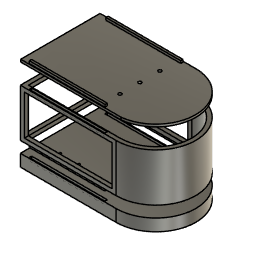
Modele3D_FusionAutodesk (Autodesk Fusion 360 design; units mm, degrees)
Autodesk Fusion 360 part; units mm, degrees
note: some values were not read from the file. Chosen so that the rebuilt part matches the saved one: which bodies a step acts on.
sketch "Esquisse1" plane through (0, 0, 0) normal (0, 0, 1) x (1, 0, 0)
  line L0 (0, 0) -> (120, 0)
  line L1 (120, 100) -> (0, 100)
  line L2 (0, 100) -> (0, 0)
  arc A0 (120, 0) -> (120, 100) centre (120, 50) ccw
  dimension "d1" = 120
  dimension "d2" = 100
  constraint horizontal L0
  constraint horizontal L1
  constraint vertical L2
  constraint coincident L0.start L2.end
  measures "d1" distance of L0.start L0.end
  measures "d2" distance of L0.start L1.end
extrude "Extrusion1" add sketch "Esquisse1" along normal blind 5 makes body 1
sketch "Esquisse2" plane through (0, 0, 5) normal (0, 0, 1) x (-1, 0, 0)
  arc A0 (-120, 0) -> (-120, -100) centre (-120, -50) ccw
  line L0 (-120, -100) -> (0, -100)
  line L1 (0, -100) -> (0, 0)
  line L2 (0, 0) -> (-120, 0)
  line L3 (-5, -95) -> (-120, -95)
  line L4 (-120, -5) -> (-5, -5)
  line L5 (-5, -5) -> (-5, -95)
  arc A1 (-120, -5) -> (-120, -95) centre (-120, -50) ccw
  dimension "d7" = 90
  constraint horizontal L3
  constraint horizontal L4
  constraint vertical L5
  constraint concentric A0 A1
  measures "d7" diameter of A1
extrude "Extrusion2" add sketch "Esquisse2" along normal blind 60 separate body makes body 2
sketch "Esquisse3" plane through (0, 0, 0) normal (0, -1, 0) x (1, 0, 0)
  line L0 (0, 5) -> (120, 5)
  line L1 (120, 5) -> (120, 65)
  line L2 (120, 65) -> (0, 65)
  line L3 (0, 65) -> (0, 5)
  line L4 (5, 60) -> (115, 60)
  line L5 (115, 60) -> (115, 10)
  line L6 (115, 10) -> (5, 10)
  line L7 (5, 10) -> (5, 60)
  constraint horizontal L4
  constraint vertical L5
  constraint horizontal L6
  constraint vertical L7
extrude "Extrusion3" cut sketch "Esquisse3" against normal blind 30 contours L4 L5 L6 L7 picked at (41.666667, 43.333333) bodies 2
sketch "Esquisse4" plane through (0, 0, 0) normal (-1, 0, 0) x (0, -1, 0)
  line L0 (-100, 5) -> (0, 5)
  line L1 (0, 5) -> (0, 65)
  line L2 (0, 65) -> (-100, 65)
  line L3 (-100, 65) -> (-100, 5)
  line L4 (-95, 60) -> (-5, 60)
  line L5 (-5, 60) -> (-5, 10)
  line L6 (-5, 10) -> (-95, 10)
  line L7 (-95, 10) -> (-95, 60)
  line L8 (-95, 60) -> (-5, 60)
  line L9 (-5, 60) -> (-5, 10)
  line L10 (-5, 10) -> (-95, 10)
  line L11 (-95, 10) -> (-95, 60)
  constraint horizontal L4
  constraint vertical L5
  constraint horizontal L6
  constraint vertical L7
  constraint horizontal L8
  constraint vertical L9
  constraint horizontal L10
  constraint vertical L11
extrude "Extrusion4" cut sketch "Esquisse4" against normal blind 30 contours L4 L5 L6 L7 L8 L9 L10 L11 picked at (-65, 43.333333) bodies 2
sketch "Esquisse5" plane through (0, 100, 0) normal (0, 1, 0) x (-1, 0, 0)
  line L0 (-120, 5) -> (0, 5)
  line L1 (0, 5) -> (0, 65)
  line L2 (0, 65) -> (-120, 65)
  line L3 (-120, 65) -> (-120, 5)
  line L4 (-115, 60) -> (-5, 60)
  line L5 (-5, 60) -> (-5, 10)
  line L6 (-5, 10) -> (-115, 10)
  line L7 (-115, 10) -> (-115, 60)
  constraint horizontal L4
  constraint vertical L5
  constraint horizontal L6
  constraint vertical L7
extrude "Extrusion5" cut sketch "Esquisse5" against normal blind 30 contours L4 L5 L6 L7 picked at (-78.333333, 43.333333) bodies 2
sketch "Esquisse6" plane through (0, 0, 65) normal (0, 0, 1) x (-1, 0, 0)
  line L0 (-120, -5) -> (-5, -5)
  line L1 (-5, -5) -> (-5, -95)
  line L2 (-5, -95) -> (-120, -95)
  arc A0 (-120, -5) -> (-120, -95) centre (-120, -50) ccw
  line L3 (0, 0) -> (-120, 0)
  arc A1 (-120, 0) -> (-120, -100) centre (-120, -50) ccw
  line L4 (-120, -100) -> (0, -100)
  line L5 (0, -100) -> (0, 0)
  line L6 (-126.00428, -0.361823) -> (0, -0.361823)
  line L7 (0, -0.361823) -> (0, -100)
  line L8 (0, -100) -> (-126.00428, -100)
  arc A2 (-125.853995, -0.361823) -> (-126.00428, -99.620223) centre (-120, -50) ccw
  line L9 (-126.00428, -100) -> (-126.00428, -99.620223)
  line L10 (-126.00428, -0.379777) -> (-126.00428, -0.361823)
  constraint concentric A0 A2
  constraint horizontal L6
  constraint vertical L7
  constraint horizontal L8
  constraint vertical L9
  constraint collinear L9 L10
extrude "Extrusion6" add sketch "Esquisse6" along normal blind 3 separate body contours L0 L1 L2 A0 picked at (-43.333333, -65) makes body 3
extrude "Extrusion7" add sketch "Esquisse6" along normal blind 3 contours A1 L4 L5 L6 L7 L8 A2 picked at (-41.666667, -98.333333) bodies 2 3
extrude "Extrusion13" add sketch "Esquisse6" along normal blind 3 separate body contours L0 L1 L2 A0 picked at (-43.333333, -65) makes body 4
extrude "Extrusion14" add sketch "Esquisse6" along normal blind 3 separate body contours A1 L4 L5 L6 L7 L8 A2 picked at (-41.666667, -98.333333) makes body 5
sketch "Esquisse7" plane through (0, 0, 68) normal (0, 0, 1) x (-1, 0, 0)
  arc A0 (-125.853995, -0.361823) -> (-126.00428, -99.620223) centre (-120, -50) ccw
  line L0 (-126.00428, -99.620223) -> (-126.00428, -99.638177)
  arc A1 (-126.00428, -99.638177) -> (-120, -100) centre (-120, -50) ccw
  line L1 (-120, -100) -> (0, -100)
  line L2 (0, -100) -> (0, -0.361823)
  line L3 (0, -0.361823) -> (-125.853995, -0.361823)
  circle A2 centre (-100, -50) radius 2
  circle A3 centre (-100, -75) radius 2
  circle A4 centre (-100, -25) radius 2
  dimension "d37" = 4
  dimension "d38" = 4
  dimension "d39" = 4
  measures "d37" diameter of A2
  measures "d38" diameter of A3
  measures "d39" diameter of A4
extrude "Extrusion15" cut sketch "Esquisse7" against normal blind 3 contours A3 picked at (-99.58434, -74.280056) bodies 2 4
extrude "Extrusion16" cut sketch "Esquisse7" against normal blind 3 contours A2 picked at (-100.880609, -50.482818) bodies 2 4
extrude "Extrusion17" cut sketch "Esquisse7" against normal blind 3 contours A4 picked at (-100.975823, -25.453448) bodies 2 4
extrude "Extrusion18" cut sketch "Esquisse7" against normal blind 3 contours A4 picked at (-100.975823, -25.453448) bodies 2 4
sketch "Esquisse9" plane through (0, 0, 0) normal (0, 0, -1) x (1, 0, 0)
  arc A0 (120, -100) -> (120, 0) centre (120, -50) ccw
  line L0 (120, 0) -> (0, 0)
  line L1 (0, 0) -> (0, -100)
  line L2 (0, -100) -> (120, -100)
  circle A1 centre (25, -25) radius 1.15
  circle A2 centre (25, -75) radius 1.15
  circle A3 centre (48.65, -25) radius 1.15
  circle A4 centre (48.65, -75) radius 1.15
  point P0 (48.65, -25)
  point P1 (48.65, -75)
  dimension "d48" = 2.3
  dimension "d51" = 23.65
  dimension "d52" = 0
  dimension "d53" = 2.3
  dimension "d56" = 23.65
  dimension "d57" = 0
  dimension "d58" = 2.3
  dimension "d59" = 2.3
  constraint coincident P0 A3.centre
  constraint coincident P1 A4.centre
  measures "d48" diameter of A1
  measures "d53" diameter of A2
  measures "d58" diameter of A3
  measures "d59" diameter of A4
move_body "Déplacer1" bodies 1 to x (1, 0, 0) y (0, 1, 0) z (0, 0, 1) at (0, 0, -25)
sketch "Esquisse10" plane through (0, 0, 5) normal (0, 0, -1) x (1, 0, 0)
  line L0 (5, -5) -> (120, -5)
  arc A0 (120, -95) -> (120, -5) centre (120, -50) ccw
  line L1 (120, -95) -> (5, -95)
  line L2 (5, -95) -> (5, -5)
  line L3 (120, 0) -> (0, 0)
  line L4 (0, 0) -> (0, -100)
  line L5 (0, -100) -> (120, -100)
  arc A1 (120, -100) -> (120, 0) centre (120, -50) ccw
  line L6 (95.000001, -98.000001) -> (20, -98.000001)
  line L7 (20, -98.000001) -> (20, -97.000001)
  line L8 (20, -97.000001) -> (95.000001, -97.000001)
  line L9 (95.000001, -97.000001) -> (95.000001, -98.000001)
  constraint horizontal L6
  constraint vertical L7
  constraint horizontal L8
  constraint vertical L9
sketch "Esquisse11" plane through (0, 0, -20) normal (0, 0, 1) x (-1, 0, 0)
  arc A0 (-120, 0) -> (-120, -100) centre (-120, -50) ccw
  line L0 (-120, -100) -> (0, -100)
  line L1 (0, -100) -> (0, 0)
  line L2 (0, 0) -> (-120, 0)
move_body "Déplacer2" bodies 1 to x (1, 0, 0) y (0, 1, 0) z (0, 0, 1) at (0, 0, 25)
hole "Perçage1" at (48.634956, 74.989415, 0) direction (0, 0, 1) diameter 2.529 depth 8 tip angle 180 bodies 1
thread "Filetage1" "ISO Metric profile 3.0 M3x0.5 6H" thread offset 0 thread depth 7.4
hole "Perçage2" at (25, 75, 0) direction (0, 0, 1) diameter 2.529 depth 8 tip angle 180 bodies 1
thread "Filetage2" "ISO Metric profile 3.0 M3x0.5 6H" thread offset 0 thread depth 7.4
hole "Perçage3" at (25.005704, 24.988017, 0) direction (0, 0, 1) diameter 2.529 depth 8 tip angle 180 bodies 1
thread "Filetage3" "ISO Metric profile 3.0 M3x0.5 6H" thread offset 0 thread depth 7.4
hole "Perçage4" at (48.67047, 24.997067, 0) direction (0, 0, 1) diameter 2.529 depth 8 tip angle 180 bodies 1
thread "Filetage4" "ISO Metric profile 3.0 M3x0.5 6H" thread offset 0 thread depth 7.4
move_body "Déplacer3" bodies 1 to x (1, 0, 0) y (0, 1, 0) z (0, 0, 1) at (0, 0, -20)
extrude "Extrusion19" add 1 faces at (96.615853, 41.81968, -15) along direction (0, 0, 1) blind 10 on bodies 1 bodies 1
sketch "Esquisse12" plane through (0, 0, -20) normal (0, 0, -1) x (1, 0, 0)
  circle A0 centre (48.67047, -24.997067) radius 1.2645
  circle A1 centre (25.005704, -24.988017) radius 1.2645
  circle A2 centre (25, -75) radius 1.2645
  circle A3 centre (48.634956, -74.989415) radius 1.2645
  arc A4 (120, -100) -> (120, 0) centre (120, -50) ccw
  line L0 (120, 0) -> (0, 0)
  line L1 (0, 0) -> (0, -100)
  line L2 (0, -100) -> (120, -100)
  circle A5 centre (145.000002, -31) radius 1.25
  circle A6 centre (145.000002, -69.000001) radius 1.25
  line L3 (114.96183, -88.38825) -> (9.547425, -88.38825)
  line L4 (9.547425, -88.38825) -> (9.547425, -86.324684)
  line L5 (9.547425, -86.324684) -> (114.96183, -86.324684)
  line L6 (114.96183, -86.324684) -> (114.96183, -88.38825)
  line L7 (118.990578, -88.38825) -> (9.845915, -88.38825)
  line L8 (9.845915, -88.38825) -> (9.845915, -86.324684)
  line L9 (9.845915, -86.324684) -> (118.990578, -86.324684)
  line L10 (118.990578, -86.324684) -> (118.990578, -88.38825)
  dimension "d83" = 2.5
  dimension "d84" = 2.5
  constraint horizontal L3
  constraint vertical L4
  constraint horizontal L5
  constraint vertical L6
  constraint horizontal L7
  constraint vertical L8
  constraint horizontal L9
  constraint vertical L10
  measures "d83" diameter of A5
  measures "d84" diameter of A6
hole "Perçage5" at (144.993119, 69.041437, -20) direction (0, 0, 1) diameter 1.875 depth 8 tip angle 180 bodies 1
thread "Filetage5" "ISO Metric profile 2.3 M2.3x0.45 6H" thread offset 0 thread depth 7.4
hole "Perçage6" at (144.947764, 30.984403, -20) direction (0, 0, 1) diameter 1.875 depth 8 tip angle 180 bodies 1
thread "Filetage6" "ISO Metric profile 2.3 M2.3x0.45 6H" thread offset 0 thread depth 7.4
move_body "Déplacer4" bodies 1 to x (1, 0, 0) y (0, 1, 0) z (0, 0, 1) at (0, 0, 5)
sketch "Esquisse13" plane through (0, 0, 5) normal (0, 0, -1) x (1, 0, 0)
  line L0 (5, -5) -> (120, -5)
  arc A0 (120, -95) -> (120, -5) centre (120, -50) ccw
  line L1 (120, -95) -> (5, -95)
  line L2 (5, -95) -> (5, -5)
  line L3 (120, 0) -> (0, 0)
  line L4 (0, 0) -> (0, -100)
  line L5 (0, -100) -> (120, -100)
  arc A1 (120, -100) -> (120, 0) centre (120, -50) ccw
  line L6 (10, -4) -> (105.000002, -4)
  line L7 (105.000002, -4) -> (105.000002, -1)
  line L8 (105.000002, -1) -> (10, -1)
  line L9 (10, -1) -> (10, -4)
  line L10 (105.000002, -96.000001) -> (10, -96.000001)
  line L11 (10, -96.000001) -> (10, -98.000001)
  line L12 (10, -98.000001) -> (105.000002, -98.000001)
  line L13 (105.000002, -98.000001) -> (105.000002, -96.000001)
  constraint horizontal L6
  constraint vertical L7
  constraint horizontal L8
  constraint vertical L9
  constraint horizontal L10
  constraint vertical L11
  constraint horizontal L12
  constraint vertical L13
extrude "Extrusion20" add sketch "Esquisse13" along normal blind 3 contours L10 L11 L12 L13 picked at (41.666667, -96.666668) bodies 2
sketch "Esquisse14" plane through (0, 0, 0) normal (0, 0, -1) x (1, 0, 0)
  line L0 (10, -99.000001) -> (105.000002, -99.000001)
  line L1 (105.000002, -99.000001) -> (105.000002, -96.000001)
  line L2 (105.000002, -96.000001) -> (10, -96.000001)
  line L3 (10, -96.000001) -> (10, -99.000001)
  line L4 (10, -1) -> (105.000002, -1)
  line L5 (105.000002, -1) -> (105.000002, -4)
  line L6 (105.000002, -4) -> (10, -4)
  line L7 (10, -4) -> (10, -1)
  constraint horizontal L0
  constraint vertical L1
  constraint horizontal L2
  constraint vertical L3
  constraint horizontal L4
  constraint vertical L5
  constraint horizontal L6
  constraint vertical L7
extrude "Extrusion21" cut sketch "Esquisse14" along normal blind 3 contours L4 L5 L6 L7 picked at (41.666667, -2) bodies 1
extrude "Extrusion22" cut sketch "Esquisse14" along normal blind 3 contours L0 L1 L2 L3 picked at (41.666667, -97.000001) bodies 1
extrude "Extrusion23" add sketch "Esquisse13" along normal blind 3 contours L6 L7 L8 L9 picked at (41.666667, -2) bodies 2
move_body "Déplacer5" bodies 1 to x (1, 0, 0) y (0, 1, 0) z (0, 0, 1) at (0, 0, -9)
combine "Combiner1" operation add target body 5 tool bodies 4
move_body "Déplacer6" bodies 5 to x (1, 0, 0) y (0, 1, 0) z (0, 0, 1) at (0, 0, 25)
ref_plane "Plan de construction2" through (85.024646, 50.180911, 65) normal (0, 0, 1) x (-1, 0, 0)
split "Scinder1" by plane through (85.024646, 50.180911, 65) normal (0, 0, 1) bodies 2 makes body 6 at (32.666667, 50.120608, 68)
move_body "Déplacer7" bodies 6 to x (1, 0, 0) y (0, 1, 0) z (0, 0, 1) at (0, 0, 15)
sketch "Esquisse15" plane through (0, 0, 65) normal (0, 0, 1) x (-1, 0, 0)
  line L0 (-5, -95) -> (-120, -95)
  arc A0 (-120, -5) -> (-120, -95) centre (-120, -50) ccw
  line L1 (-120, -5) -> (-5, -5)
  line L2 (-5, -5) -> (-5, -95)
  line L3 (0, -100) -> (0, 0)
  line L4 (0, 0) -> (-120, 0)
  arc A1 (-120, 0) -> (-120, -100) centre (-120, -50) ccw
  line L5 (-120, -100) -> (0, -100)
  line L6 (-10, -4) -> (-105.000002, -4)
  line L7 (-105.000002, -4) -> (-105.000002, -1)
  line L8 (-105.000002, -1) -> (-10, -1)
  line L9 (-10, -1) -> (-10, -4)
  line L10 (-10, -99.000001) -> (-105.000002, -99.000001)
  line L11 (-105.000002, -99.000001) -> (-105.000002, -96.000001)
  line L12 (-105.000002, -96.000001) -> (-10, -96.000001)
  line L13 (-10, -96.000001) -> (-10, -99.000001)
  constraint horizontal L6
  constraint vertical L7
  constraint horizontal L8
  constraint vertical L9
  constraint horizontal L10
  constraint vertical L11
  constraint horizontal L12
  constraint vertical L13
extrude "Extrusion24" cut sketch "Esquisse15" against normal blind 3 contours L6 L7 L8 L9 picked at (-41.666667, -3) bodies 2
extrude "Extrusion25" cut sketch "Esquisse15" against normal blind 3 contours L10 L11 L12 L13 picked at (-41.666667, -98.000001) bodies 2
sketch "Esquisse18" plane through (0, 0, 93) normal (0, 0, 1) x (-1, 0, 0)
  circle A0 centre (-100, -75) radius 2
  circle A1 centre (-100, -50) radius 2
  circle A2 centre (-100, -25) radius 2
  arc A3 (-125.853995, -0.361823) -> (-126.00428, -99.620223) centre (-120, -50) ccw
  line L0 (-126.00428, -99.620223) -> (-126.00428, -99.638177)
  arc A4 (-126.00428, -99.638177) -> (-120, -100) centre (-120, -50) ccw
  line L1 (-120, -100) -> (0, -100)
  line L2 (0, -100) -> (0, -0.361823)
  line L3 (0, -0.361823) -> (-125.853995, -0.361823)
  line L4 (-105.000002, -99.000001) -> (-10.950002, -99.000001)
  line L5 (-10.950002, -99.000001) -> (-10.950002, -96.227532)
  line L6 (-10.950002, -96.227532) -> (-105.000002, -96.227532)
  line L7 (-105.000002, -96.227532) -> (-105.000002, -99.000001)
  line L8 (-105.000002, -4) -> (-9.930002, -4)
  line L9 (-9.930002, -4) -> (-9.930002, -1.165732)
  line L10 (-9.930002, -1.165732) -> (-105.000002, -1.165732)
  line L11 (-105.000002, -1.165732) -> (-105.000002, -4)
  dimension "d108" = 94.05
  dimension "d109" = 95.07
  constraint horizontal L4
  constraint vertical L5
  constraint horizontal L6
  constraint vertical L7
  constraint horizontal L8
  constraint vertical L9
  constraint horizontal L10
  constraint vertical L11
extrude "Extrusion26" add sketch "Esquisse18" along normal blind 3 contours L8 L9 L10 L11 picked at (-73.310002, -2.110488) bodies 5
extrude "Extrusion27" add sketch "Esquisse18" along normal blind 3 contours L4 L5 L6 L7 picked at (-73.650002, -97.151689) bodies 5
delete_body "RemoveBody1" bodies 6
move_body "Déplacer8" [suppressed]
